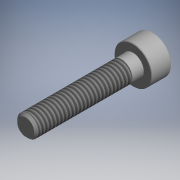
# Autodesk Inventor part: DIN-912 - M4x20(F)
Saved by Autodesk Inventor 2017.3 (Build 213256000, 256)
## iProperties
Part Number: DIN-912 - M4x20(F)
Material: Generic
Catalog Web Link: www.cadenas.de
Description: DIN-912-Cylinder screw
Vendor: FESTO
Document SubType Name: Modeling
Designer: partserver
Manufacturer: FESTO
Mass: 0.3848 g
Surface Area: 4.26651 cm^2
Volume: 0.3848 cm^3
Density: 1 g/cm^3
Appearance: PSOLRGB-192-192-192
Category: PARTsolutions
Company: FESTO
Title: DIN-912 - M4x20(F)
Author: Cadenas PARTsolutions
Comments: Cylinder screw
PSOL_IDENT_0: {$CADENAS_DATA\23d-libs\festo\zyl_zubeh\d912\din_912.prj},178 {VTYP=3D},{NB=DIN-912 - M4x20(F)},{LIN
PSOL_IDENT_1: A=DIN-912 - M4x20(F)},{NN=DIN-912},{DATE=01.07.2020 05:33:41},{GEOMDATE=01.07.2020 05:33:34},{VERSIO
PSOL_IDENT_2: N=},{LINEID=240},{WBVAR=},{WBNUMERIC=}  {NB=DIN-912 - M4x20(F)},{LINA=DIN-912 - M4x20(F)},{KT=X},{ID
PSOL_IDENT_3: NR=},{GEW=M4},{DG=4.000},{P=0.700},{L=20.000},{B=20.000},{FORM=1},{GKD=3.141},{DK=7.000},{DADIN=4.70
PSOL_IDENT_4: 0},{DS=4.000},{E=3.440},{LF=0.600},{K=4.000},{R=0.200},{S=3.000},{T=2.000},{V=0.400},{DW=6.530},{W=1
PSOL_IDENT_5: .400},{NENN=M4x20},{DA=4.1},{BL=17.9}
NB: DIN-912 - M4x20(F)
NN: DIN-912
NT: Cylinder screw
NBSYN: DIN-912 - $NENN.(F)
LINA: DIN-912 - M4x20(F)
CATALOG: Festo
ROWDESC: M4x20
GEW: M4
DG: 4
P: 0.7
L: 20
B: 20
FORM: 1
GKD: 3.141
DK: 7
DADIN: 4.7
DS: 4
E: 3.44
LF: 0.6
K: 4
R: 0.2
S: 3
T: 2
V: 0.4
DW: 6.53
W: 1.4
SUPPLIER: FESTO
ARTICLENO: DIN-912 - M4x20(F)
BOMINFO: DIN-912 - M4x20(F)
CREATOR: CADENAS GmbH
Autodesk Inventor part; units mm, degrees
sketch "Sketch_1" plane through (0, 0, 0) normal (0, 0, 1) x (1, 0, 0)
  line L0 (0, -20) -> (0, 4)
  line L1 (0, 1.134) -> (1.5, 2)
  line L2 (1.5, 2) -> (1.5, 3.7679)
  line L3 (1.5, 3.7679) -> (1.7321, 4)
  line L4 (1.7321, 4) -> (3.1, 4)
  line L5 (3.1, 4) -> (3.5, 3.6)
  line L6 (3.5, 3.6) -> (3.5, 0.1)
  line L7 (3.5, 0.1) -> (3.4, 0)
  line L8 (3.4, 0) -> (2.05, 0)
  line L9 (2.05, 0) -> (2, -0.6)
  line L10 (2, -0.6) -> (2, -19.5705)
  line L11 (2, -19.5705) -> (1.5705, -20)
  line L12 (1.5705, -20) -> (0, -20)
  line L13 (0, -20) -> (0, 1.134)
  constraints: 28 end point
revolve "Revolution1" add sketch "Sketch_1" angle 360 about axis through (0, -20, 0) along (0, -1, 0)
thread "Thread1" size "M4x0.7" class "6g" standard "ISO Metric profile" length 17.4705
sketch "Sketch_2" plane through (0, 4, 0) normal (0, 1, 0) x (1, 0, 0)
  line L0 (-1.5, -0.866) -> (0, -1.7321)
  line L1 (0, -1.7321) -> (1.5, -0.866)
  line L2 (1.5, -0.866) -> (1.5, 0.866)
  line L3 (1.5, 0.866) -> (0, 1.7321)
  line L4 (0, 1.7321) -> (-1.5, 0.866)
  line L5 (-1.5, 0.866) -> (-1.5, -0.866)
  constraints: 12 end point
extrude "Extrusion1" cut sketch "Sketch_2" against normal blind 2
ref_plane "ANBAU_XY" through (0, 0, 0) normal (0, 1, 0) x (1, 0, 0)
ref_plane "ANBAU_YZ" through (0, 0, 0) normal (1, 0, 0) x (0, 0, -1)
ref_plane "ANBAU_ZX" through (0, 0, 0) normal (0, 0, -1) x (0, 1, 0)
ref_plane "Schraube_XY" through (0, 0, 0) normal (0, 1, 0) x (1, 0, 0)
ref_plane "Schraube_YZ" through (0, 0, 0) normal (1, 0, 0) x (0, 0, -1)
ref_plane "Schraube_ZX" through (0, 0, 0) normal (0, 0, -1) x (0, 1, 0)
ref_plane "insert_XY" through (0, 0, 0) normal (0, 1, 0) x (1, 0, 0)
ref_plane "insert_YZ" through (0, 0, 0) normal (1, 0, 0) x (0, 0, -1)
ref_plane "insert_ZX" through (0, 0, 0) normal (0, 0, -1) x (0, 1, 0)
ref_plane "schrauben_punkt_XY" through (0, -20, 0) normal (0, 1, 0) x (1, 0, 0)
ref_plane "schrauben_punkt_YZ" through (0, -20, 0) normal (1, 0, 0) x (0, 0, -1)
ref_plane "schrauben_punkt_ZX" through (0, -20, 0) normal (0, 0, -1) x (0, 1, 0)
body "Solid1"
